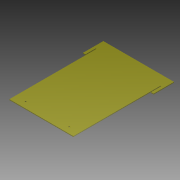
# Autodesk Inventor part: door
Saved by Autodesk Inventor 2014 SP2 (Build 180246200, 246)
## iProperties
Created: 2016-05-06
Part Number: door
Material: Generic
Document SubType Name: Modeling
Designer: cruiser
Density: 1 g/cm^3
Appearance: Clear - Yellow
Author: cruiser
Autodesk Inventor part; units mm, degrees
ref_plane "YZ Plane" through (0, 0, 0) normal (1, 0, 0) x (0, 1, 0)
ref_plane "XZ Plane" through (0, 0, 0) normal (0, 1, 0) x (-1, 0, 0)
ref_plane "XY Plane" through (0, 0, 0) normal (0, 0, 1) x (1, 0, 0)
sketch "Sketch1" plane through (0, 0, 0) normal (0, 0, 1) x (1, 0, 0)
  line L0 (125.5, -166.9563) -> (-125.5, -166.9563)
  line L1 (-125.5, -166.9563) -> (-125.5, 166.9563)
  line L2 (-125.5, 166.9563) -> (125.5, 166.9563)
  line L3 (125.5, 166.9563) -> (125.5, -166.9563)
  line L4 (125.5, -166.9563) -> (-125.5, 166.9563) construction
  line L5 (-125.5, -166.9563) -> (125.5, 166.9563) construction
  line L6 (-125.5, -166.9563) -> (125.5, -166.9563)
  line L7 (125.5, -166.9563) -> (125.5, -214.9563)
  line L8 (125.5, -214.9563) -> (-125.5, -214.9563)
  line L9 (-125.5, -214.9563) -> (-125.5, -166.9563)
  point P0 (0, 0)
  dimension "d0" = 251
  dimension "d1" = 333.9125
  dimension "d4" = 48
  dimension "d5" = 0
  dimension "d6" = 0
  constraints: 20 end point, 4 parallel, 2 horizontal, 2 midpoint, 2 perpendicular, 1 point on line
  measures "d0" distance of L1.end L2.end
  measures "d1" distance of L0.end L1.end
  measures "d4" distance of L6.end L7.end
  measures "d5" distance between parallel lines of L1 L9
  measures "d6" distance between parallel lines of L3 L7
extrude "Extrusion1" add sketch "Sketch1" along normal blind 3.15
sketch "Sketch2" plane through (0, 0, 3.15) normal (0, 0, 1) x (1, 0, 0)
  line L0 (125.5, 166.9563) -> (-125.5, 166.9563) projected
  line L1 (-125.5, 166.9563) -> (-138.65, 166.9563)
  line L2 (-138.65, 166.9563) -> (-138.65, 86.9563)
  line L3 (-138.65, 86.9563) -> (-125.5, 86.9563)
  line L4 (-125.5, 86.9563) -> (-125.5, 166.9563)
  line L5 (-125.5, 86.9563) -> (-128.65, 86.9563)
  line L6 (-128.65, 86.9563) -> (-128.65, 126.9563)
  line L7 (-128.65, 126.9563) -> (-125.5, 126.9563)
  line L8 (-125.5, 126.9563) -> (-125.5, 86.9563)
  line L9 (0, 166.9563) -> (0, 0)
  line L10 (125.5, 166.9563) -> (138.65, 166.9563)
  line L11 (138.65, 166.9563) -> (138.65, 86.9563)
  line L12 (138.65, 86.9563) -> (125.5, 86.9563)
  line L13 (125.5, 86.9563) -> (125.5, 166.9563)
  line L14 (125.5, 86.9563) -> (128.65, 86.9563)
  line L15 (128.65, 86.9563) -> (128.65, 126.9563)
  line L16 (128.65, 126.9563) -> (125.5, 126.9563)
  line L17 (125.5, 126.9563) -> (125.5, 86.9563)
  dimension "d7" = 80
  dimension "d8" = 13.15
  dimension "d9" = 3.15
  dimension "d10" = 40
  constraints: 34 end point, 6 symmetric about line, 5 parallel, 2 horizontal, 2 perpendicular, 1 midpoint
  measures "d7" distance of L1.end L2.end
  measures "d8" distance of L0.end L1.end
  measures "d9" distance of L6.end L7.end
  measures "d10" distance between parallel lines of L1 L7
extrude "Extrusion2" add sketch "Sketch2" against normal blind 3.15 contours L4 L7 L6 L3 L2 L1 | L10 L11 L12 L15 L16 L13
sketch "Sketch3" plane through (0, 0, 3.15) normal (0, 0, 1) x (1, 0, 0)
  line L0 (-125.5, -214.9563) -> (125.5, -214.9563) projected
  circle A0 centre (-85.7667, -190.9563) radius 2.5
  line L1 (0, 0) -> (0, -214.9563)
  circle A1 centre (85.7667, -190.9563) radius 2.5
  dimension "d13" = 5
  dimension "d14" = 24
  dimension "d15" = 85.7667
  constraints: 2 centre point, 2 end point, 1 midpoint, 1 symmetric about line, 1 other
  measures "d13" diameter of A0
  measures "d14" distance from line of L0 A0.centre
  measures "d15" distance from line of L1 A0.centre
extrude "Extrusion3" cut sketch "Sketch3" against normal blind 10
equation "\"d0\" = door_x"
equation "\"d1\" = door_z"
equation "\"d4\" = door_overlap"
equation "\"d2\" = clear_acrylic"
equation "\"d7\" = protection_slot_length"
equation "\"d8\" = protection_slot_width + clear_acrylic"
equation "\"d9\" = clear_acrylic"
equation "\"d10\" = 0.5 * protection_slot_length"
equation "\"d11\" = clear_acrylic"
equation "\"d13\" = m5_diameter"
equation "\"d14\" = 0.5 * door_overlap"
equation "\"d15\" = 0.333333 * drawer_x"
equation "\"sm_thickness\" = 1.5875"
equation "\"very_thick_acrylic\" = 9.45"
equation "\"thick_acrylic\" = 5.88"
equation "\"thin_acrylic\" = 3.15"
equation "\"clear_acrylic\" = 3.15"
equation "\"wood_thickness\" = 6.72"
equation "\"m3_diameter\" = 3"
equation "\"m4_diameter\" = 4"
equation "\"m5_diameter\" = 5"
equation "\"brass_insert_drill\" = 4"
equation "\"m5_brass_insert_drill\" = 6.7"
equation "\"m3_main_length\" = 14"
equation "\"m3_main_nut_width\" = 5.7"
equation "\"m3_main_nut_thickness\" = 2.5"
equation "\"m3_main_extra\" = 1"
equation "\"stepper_screw_space\" = 35"
equation "\"stepper_shaft_diameter\" = 5"
equation "\"stepper_body_diameter\" = 28"
equation "\"laser_body_diameter\" = 12"
equation "\"carrier_y\" = 251"
equation "\"carrier_z\" = 12"
equation "\"visor_x\" = 257.3"
equation "\"visor_y\" = 111.0625"
equation "\"protection_slot\" = 44.2"
equation "\"protection_slot_offset\" = 55.25"
equation "\"protection_slot_length\" = 80"
equation "\"window_z\" = 333.9125"
equation "\"window_y\" = 92.0625"
equation "\"window_overlap\" = 48"
equation "\"door_x\" = 251"
equation "\"door_z\" = 333.9125"
equation "\"door_sensor\" = 35"
equation "\"reservoir_x\" = 201"
equation "\"reservoir_y\" = 201"
equation "\"linear_bearing_spacing\" = 271"
equation "\"motor_spacing\" = 337"
equation "\"tray_border\" = 25"
equation "\"tray_x\" = 251"
equation "\"tray_y\" = 251"
equation "\"bed_z\" = 25"
equation "\"crane_z2\" = 12"
equation "\"end_stop_spacing\" = 19"
equation "\"door_overlap\" = 48"
equation "\"acrylic_into_frame\" = 5"
equation "\"protection_slot_width\" = 10"
equation "\"frame_top_z\" = 385"
equation "\"nema17_x\" = 43"
equation "\"drawer_z_from_bottom\" = 25"
equation "\"laser_diameter\" = 12"
equation "\"t_galvo_frame\" = 6.72"
equation "\"laser_z\" = 75"
equation "\"drawer_y\" = 88.65"
equation "\"laser_y\" = 15"
equation "\"subframe_x\" = 195"
equation "\"galvo_frame_z\" = 65"
equation "\"subframe_y_offset\" = 27.5"
equation "\"drawer_x\" = 257.3"
equation "\"printer_z\" = 289"
equation "\"lcd_x\" = 72"
equation "\"frame_tilt\" = 1deg"
equation "\"frame_foot_z\" = 12"
equation "\"frame_border\" = 46.35"
equation "\"frame_bottom_z\" = 275"
equation "\"z_min_from_center\" = 115"
equation "\"thumb_nut_diameter\" = 7"
equation "\"laser_z_offset\" = 55"
equation "\"laser_y_offset\" = 19.4"
equation "\"thumb_nut_offset_y\" = 0"
equation "\"galvo_frame_y_offset\" = 27.5"
equation "\"frame_total_z\" = 661.5875"
equation "\"galvo_frame_x\" = 66"
equation "\"drawer_z\" = 278.175"
equation "\"lcd_y\" = 25"
equation "\"m3_press_nut_drill\" = 4.5"
equation "\"m3_head\" = 6"
equation "\"m5_press_nut_drill\" = 6.5"
equation "\"drawer_support_from_top\" = 48"
equation "\"laser_gap\" = 1"
equation "\"frame_screw_from_center\" = 25"
equation "\"drawer_screw_from_center\" = 54"
equation "\"frame_face_y\" = 44"
equation "\"switch_spacing\" = 19"
body "Solid1"
